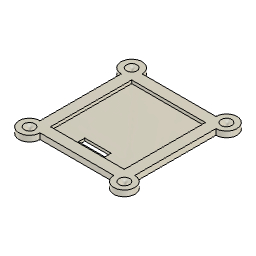
keypad_holder (Autodesk Fusion 360 design; units mm, degrees)
Autodesk Fusion 360 part; units mm, degrees
sketch "Sketch1" plane through (0, 0, 0) normal (0, 0, 1) x (1, 0, 0)
  line L0 (0, 0) -> (70, 0)
  line L1 (70, 0) -> (70, 77)
  line L2 (70, 77) -> (0, 77)
  line L3 (0, 77) -> (0, 0)
  dimension "d1" = 70
  dimension "d2" = 77
  constraint horizontal L0
  constraint vertical L1
  constraint horizontal L2
  constraint vertical L3
  constraint coincident L0.start L3.end
  measures "d1" distance of L0.start L0.end
  measures "d2" distance of L0.start L2.end
extrude "Extrude1" add sketch "Sketch1" along normal blind 1 makes body 1
copy_body "Body->Comp1" bodies 1 removing the originals makes body 2 in component "KeyPad"
sketch "Sketch2" plane through (0, 0, 1) normal (0, 0, 1) x (-1, 0, 0)
  line L0 (0, -77) -> (0, 0)
  line L1 (0, 0) -> (-70, 0)
  line L2 (-70, 0) -> (-70, -77)
  line L3 (-70, -77) -> (0, -77)
  line L4 (-70, 0) -> (-35, 0)
  line L5 (-35, 0) -> (-35, -2)
  line L6 (-35, -2) -> (-47.5, -2)
  line L7 (-47.5, -2) -> (-47.5, -12)
  line L8 (-47.5, -12) -> (-35, -12)
  line L9 (-35, -12) -> (-35, -2)
  line L10 (-35, -2) -> (-22.5, -2)
  line L11 (-22.5, -2) -> (-22.5, -12)
  line L12 (-22.5, -12) -> (-35, -12)
  line L13 (-35, -12) -> (-35, -2)
  line L14 (-37, -4) -> (-45.5, -4)
  line L15 (-45.5, -4) -> (-45.5, -10)
  line L16 (-45.5, -10) -> (-37, -10)
  line L17 (-37, -10) -> (-37, -4)
  line L18 (-47.5, -4) -> (-22.5, -4)
  line L19 (-22.5, -4) -> (-22.5, -10)
  line L20 (-22.5, -10) -> (-47.5, -10)
  line L21 (-47.5, -10) -> (-47.5, -4)
  dimension "d26" = 2
  dimension "d27" = 12.5
  dimension "d28" = 10
  dimension "d29" = 10
  dimension "d30" = -2
  dimension "d31" = 6
  constraint coincident L1.end L2.start
  constraint midpoint L1 L4.end
  constraint perpendicular L1 L5
  constraint horizontal L6
  constraint vertical L7
  constraint horizontal L8
  constraint vertical L9
  constraint horizontal L10
  constraint vertical L11
  constraint horizontal L12
  constraint vertical L13
  constraint horizontal L18
  constraint vertical L19
  constraint horizontal L20
  constraint vertical L21
  constraint coincident L7 L18.start
  measures "d26" distance of L4.end L5.end
  measures "d27" distance of L5.end L6.end
  measures "d28" distance of L5.end L8.end
  measures "d29" distance of L5.end L8.end
  measures "d31" distance of L18.start L20.end
sketch "Sketch3" plane through (0, 0, 0) normal (0, 0, -1) x (1, 0, 0)
  line L0 (0, 0) -> (0, -77)
  line L1 (0, -77) -> (70, -77)
  line L2 (70, -77) -> (70, 0)
  line L3 (70, 0) -> (0, 0)
  line L4 (80, -87) -> (80, 10)
  line L5 (80, 10) -> (-10, 10)
  line L6 (-10, 10) -> (-10, -87)
  line L7 (-10, -87) -> (80, -87)
  dimension "d5" = 10
extrude "Extrude1'" add sketch "Sketch3" against normal blind 3 separate body makes body 3 in component "BackPlate"
sketch "Sketch4" plane through (0, 0, 0) normal (0, 0, -1) x (1, 0, 0)
  line L0 (0, 0) -> (70, 0)
  line L1 (70, 0) -> (70, -77)
  line L2 (70, -77) -> (0, -77)
  line L3 (0, -77) -> (0, 0)
  line L4 (-10, -87) -> (80, -87)
  line L5 (80, -87) -> (80, 10)
  line L6 (80, 10) -> (-10, 10)
  line L7 (-10, 10) -> (-10, -87)
extrude "Extrude2" add sketch "Sketch4" along normal blind 2.5 contours L0 L1 L2 L3 | L4 L5 L6 L7 bodies 3 in component "BackPlate"
sketch "Sketch5" plane through (0, 0, -2.5) normal (0, 0, -1) x (1, 0, 0)
  line L0 (-10, 10) -> (-10, -87)
  line L1 (-10, -87) -> (80, -87)
  line L2 (80, -87) -> (80, 10)
  line L3 (80, 10) -> (-10, 10)
  circle A0 centre (80, 10) radius 10
  circle A1 centre (-10, 10) radius 10
  circle A2 centre (-10, -87) radius 10
  circle A3 centre (80, -87) radius 10
  dimension "d10" = 20
  dimension "d11" = 20
  dimension "d12" = 20
  dimension "d13" = 20
  constraint coincident L2.end L3.start
  constraint coincident L0.start L3.end
  constraint coincident L0.end L1.start
  constraint coincident L1.end L2.start
  measures "d10" diameter of A0
  measures "d11" diameter of A1
  measures "d12" diameter of A2
  measures "d13" diameter of A3
extrude "Extrude3" add sketch "Sketch5" against normal blind 5.5 contours L0 L3 A1 | L0 L1 A2 | L2 L3 A0 | L1 L2 A3 picked at (-10.4891, 3.3694) picked at (-14.8152, -82.4155) picked at (75.4782, 14.8733) picked at (73.3706, -87.4968) bodies 3 in component "BackPlate"
sketch "Sketch6" plane through (0, 0, 3) normal (0, 0, 1) x (-1, 0, 0)
  line L0 (-70, 0) -> (0, 0)
  line L1 (0, 0) -> (0, -77)
  line L2 (0, -77) -> (-70, -77)
  line L3 (-70, -77) -> (-70, 0)
  line L4 (-70, -87) -> (0, -87)
  arc A0 (0, -87) -> (10, -77) centre (10, -87) ccw
  line L5 (10, -77) -> (10, 0)
  arc A1 (10, 0) -> (0, 10) centre (10, 10) ccw
  line L6 (0, 10) -> (-70, 10)
  arc A2 (-70, 10) -> (-80, 0) centre (-80, 10) ccw
  line L7 (-80, 0) -> (-80, -77)
  arc A3 (-80, -77) -> (-70, -87) centre (-80, -87) ccw
  circle A4 centre (10, 10) radius 1
  circle A5 centre (-80, 10) radius 1
  circle A6 centre (10, -87) radius 1
  circle A7 centre (-80, -87) radius 1
  dimension "d16" = 2
  dimension "d19" = -90
  dimension "d20" = -97
  constraint concentric A1 A4
  measures "d16" diameter of A4
extrude "Extrude4" cut sketch "Sketch6" against normal blind 5.5 contours A4 | A5 | A6 | A7 bodies 3 in component "BackPlate"
sketch "Sketch7" plane through (0, 0, 3) normal (0, 0, 1) x (-1, 0, 0)
  circle A0 centre (-80, -87) radius 1
  circle A1 centre (-80, 10) radius 1
  circle A2 centre (10, -87) radius 1
  circle A3 centre (10, 10) radius 1
  line L0 (-70, 0) -> (0, 0)
  line L1 (0, 0) -> (0, -77)
  line L2 (0, -77) -> (-70, -77)
  line L3 (-70, -77) -> (-70, 0)
  line L4 (-70, -87) -> (0, -87)
  arc A4 (0, -87) -> (10, -77) centre (10, -87) ccw
  line L5 (10, -77) -> (10, 0)
  arc A5 (10, 0) -> (0, 10) centre (10, 10) ccw
  line L6 (0, 10) -> (-70, 10)
  arc A6 (-70, 10) -> (-80, 0) centre (-80, 10) ccw
  line L7 (-80, 0) -> (-80, -77)
  arc A7 (-80, -77) -> (-70, -87) centre (-80, -87) ccw
  circle A8 centre (10, 10) radius 4
  dimension "d23" = 8
  constraint concentric A3 A8
  measures "d23" diameter of A8
fillet "Fillet1" radius 4 4 edges at (80.9323, -10.3616, 3) (-9.0677, 86.6384, 3) (80.9323, 86.6384, 3) (-9.0677, -10.3616, 3) on bodies 3 in component "BackPlate"
extrude "Extrude1''" cut sketch "Sketch2" against normal blind 10 contours L9 L11 L13 L18 L19 L20 | L9 L13 L17 L18 L20 | L7 L15 L18 L20 L21 | L14 L15 L16 L17 L18 L20 bodies 2 in component "KeyPad"
extrude "Extrude5" cut sketch "Sketch2" against normal blind 10 contours L9 L11 L13 L18 L19 L20 | L9 L13 L17 L18 L20 | L7 L15 L18 L20 L21 | L14 L15 L16 L17 L18 L20 bodies 3 in component "BackPlate"
component "KeyPad" placed x (1, 0, 0) y (0, 1, 0) z (0, 0, 1) at (0, 0, 0)
component "BackPlate" placed x (1, 0, 0) y (0, 1, 0) z (0, 0, 1) at (0, 0, 0)
